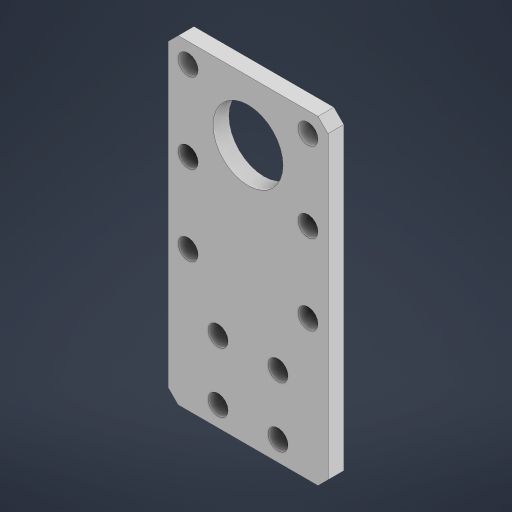
# Autodesk Inventor part: ArmSidePlate
Saved by Autodesk Inventor 2024 (Build 280153000, 153)
## iProperties
Created: 2023-10-19
Part Number: ArmSidePlate
Material: Generic
Document SubType Name: Modeling
Designer: avsar
Density: 1 g/cm^3
Appearance: Default
Author: avsar
Autodesk Inventor part; units mm, degrees
ref_plane "YZ Plane" through (0, 0, 0) normal (1, 0, 0) x (0, 1, 0)
ref_plane "XZ Plane" through (0, 0, 0) normal (0, 1, 0) x (-1, 0, 0)
ref_plane "XY Plane" through (0, 0, 0) normal (0, 0, 1) x (1, 0, 0)
sketch "Sketch1" plane through (0, 0, 0) normal (0, 0, 1) x (1, 0, 0)
  line L0 (16, -32) -> (-16, -32)
  line L1 (-16, -32) -> (-16, 32)
  line L2 (-16, 32) -> (16, 32)
  line L3 (16, 32) -> (16, -32)
  line L4 (16, -32) -> (-16, 32) construction
  line L5 (-16, -32) -> (16, 32) construction
  circle A0 centre (0, -22) radius 2.5 construction
  circle A1 centre (-6, -28) radius 2
  circle A2 centre (6, -28) radius 2
  circle A3 centre (6, -16) radius 2
  circle A4 centre (-6, -16) radius 2
  line L6 (-16, 0) -> (16, 0) construction
  point P0 (0, 0)
  point P1 (0, -32)
  dimension "d0" = 32
  dimension "d1" = 64
  dimension "d2" = 5
  dimension "d3" = 10
  dimension "d4" = 4
  dimension "d5" = 6
  dimension "d6" = 6
  dimension "d9" = 360
  constraints: 14 end point, 5 centre point, 5 midpoint, 2 parallel, 1 horizontal, 1 perpendicular, 1 vertical alignment, 9 other
  measures "d0" distance of L1.end L2.end
  measures "d1" distance of L0.end L1.end
  measures "d2" diameter of A0
  measures "d3" distance of point (0, -32) A0.centre
  measures "d4" diameter of A1
  measures "d5" horizontal distance of A0.centre A1.centre
  measures "d6" horizontal distance of A0.centre A1.centre
extrude "Extrusion1" add sketch "Sketch1" along normal mid plane 3.175
sketch "Sketch2" plane through (0, 0, 1.5875) normal (0, 0, 1) x (1, 0, 0)
  line L0 (16, 32) -> (-16, 32) construction
  line L1 (-16, 32) -> (-16, -32) construction
  line L2 (-16, -32) -> (16, -32) construction
  line L3 (16, -32) -> (16, 32) construction
  circle A0 centre (-6, -16) radius 2 construction
  circle A1 centre (6, -16) radius 2 construction
  circle A2 centre (6, -28) radius 2 construction
  circle A3 centre (-6, -28) radius 2 construction
  circle A4 centre (0, 20) radius 7
  circle A5 centre (-12, 28) radius 2
  line L4 (0, 32) -> (0, -32) construction
  line L5 (-16, 32) -> (-16, -32) projected
  line L6 (-16, 0) -> (16, 0) construction
  circle A6 centre (-12, 12) radius 2
  circle A7 centre (-12, -4) radius 2
  circle A8 centre (12, 28) radius 2
  circle A9 centre (12, 12) radius 2
  circle A10 centre (12, -4) radius 2
  point P0 (0, 0)
  dimension "d14" = 14
  dimension "d15" = 20
  dimension "d16" = 4
  dimension "d17" = 4
  dimension "d18" = 4
  dimension "d19" = 4
  dimension "d20" = 16
  dimension "d21" = 4
  dimension "d22" = 16
  constraints: 7 centre point, 4 end point, 4 midpoint, 3 symmetric about line, 3 vertical alignment, 3 other
  measures "d14" diameter of A4
  measures "d15" distance of point (0, 0) A4.centre
  measures "d16" diameter of A5
  measures "d17" distance from line of L0 A5.centre
  measures "d18" distance from line of L1 A5.centre
  measures "d19" diameter of A6
  measures "d20" distance of A5.centre A6.centre
  measures "d21" diameter of A7
  measures "d22" distance of A6.centre A7.centre
extrude "Extrusion2" cut sketch "Sketch2" against normal through all
chamfer "Chamfer1" distance 2 angle 45 4 edges at (16, 32, 0) (-16, 32, 0) (16, -32, 0) (-16, -32, 0)
body "Solid1"
